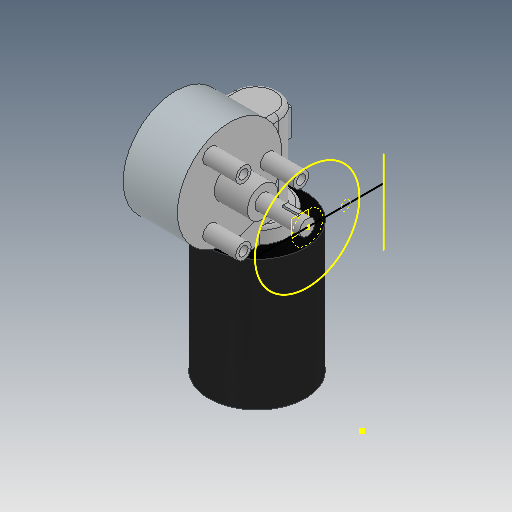
# Autodesk Inventor part: motor
Saved by Autodesk Inventor 2025.2 (Build 292293000, 293)
## iProperties
Created: 2024-10-20
Part Number: motor
Material: ABS Plastic
Document SubType Name: Modeling
Designer: email
Density: 1.06 g/cm^3
Appearance: Zinc
Author: email
Autodesk Inventor part; units mm, degrees
ref_plane "XZ Plane" through (0, 0, 0) normal (0, 1, 0) x (-1, 0, 0)
sketch "Sketch1" plane through (0, 0, 0) normal (0, 1, 0) x (-1, 0, 0)
  circle A0 centre (0, 0) radius 31.5
  circle A1 centre (0, 0) radius 20
  dimension "d0" = 63
  dimension "d29" = 40
  constraints: 2 centre point, 2 coincident
  measures "d0" diameter of A0
  measures "d29" diameter of A1
extrude "Extrusion1" add sketch "Sketch1" along normal blind 85 contours A0 | A1
sketch "Sketch2" plane through (0, 0, 0) normal (1, 0, 0) x (0, 1, 0)
  line L0 (0, -31.5) -> (85, -31.5) projected
  line L1 (0, -31.5) -> (0, 69.5)
  line L2 (0, 69.5) -> (166.6, 69.5)
  line L3 (166.6, 69.5) -> (166.6, 35.5)
  line L4 (166.6, 35.5) -> (132.6, 35.5)
  circle A0 centre (132.6, 35.5) radius 34
  circle A1 centre (132.6, 35.5) radius 25
  circle A2 centre (132.6, 10.5) radius 5
  circle A3 centre (132.6, 10.5) radius 3
  circle A4 centre (154.2506, 48) radius 5
  circle A5 centre (154.2506, 48) radius 3
  circle A6 centre (110.9494, 48) radius 5
  circle A7 centre (110.9494, 48) radius 3
  line L5 (85, -31.5) -> (85, 31.5) projected
  line L6 (85, 25.7084) -> (151.9419, 25.7084)
  line L7 (151.9419, 25.7084) -> (151.9419, -14.2916)
  line L8 (151.9419, -14.2916) -> (85, -14.2916)
  line L9 (85, -14.2916) -> (85, 25.7084)
  circle A8 centre (132.6, 35.5) radius 10
  circle A9 centre (132.6, 35.5) radius 5
  line L10 (85, 31.5) -> (85, 0)
  line L11 (85, 0) -> (100.814, 0)
  point P0 (0, 0)
  point P1 (151.9419, 7.5377)
  point P2 (134.9384, 1.5805)
  point P3 (130.2616, 1.5805)
  point P4 (100.0404, 25.7084)
  point P5 (92.907, 0)
  dimension "d8" = 50
  dimension "d3" = 101
  dimension "d4" = 166.6
  dimension "d5" = 34
  dimension "d6" = 34
  dimension "d7" = 68
  dimension "d9" = 10
  dimension "d10" = 6
  dimension "d13" = 360
  dimension "d21" = 20
  dimension "d22" = 10
  dimension "d26" = 40
  dimension "d49" = 69.5
  dimension "d50" = 35.5
  constraints: 20 end point, 9 centre point, 7 coincident, 3 horizontal, 3 point on line, 2 parallel, 2 perpendicular, 2 vertical, 1 midpoint, 1 vertical alignment, 15 other
  measures "d3" distance of L1.start L1.end
  measures "d4" distance of L1.end L2.end
  measures "d5" distance of L2.end L3.end
  measures "d6" distance of L3.end L4.end
  measures "d7" diameter of A0
  measures "d9" diameter of A2
  measures "d10" diameter of A3
  measures "d21" diameter of A8
  measures "d22" diameter of A9
  measures "d26" distance of L6.end L7.end
  measures "d49" distance between parallel lines of L2 L11
  measures "d50" distance from line of point (92.907, 0) L4
extrude "Extrusion2" add sketch "Sketch2" along normal mid plane 30 contours L5 L6 A0 L7 L8 | A0 L4 A1 A4 A6 L6 | A0 L7 A1 L4 | L6 A1 A2 L7 A0 | A1 L7 L6 A8 L4 | L4 A8 L6 A1 A6 A4 | L6 A8 L7 A1 A2 | A8 L6 | A4 A1 A5 | A1 A5 A4 | A6 A1 A7 | A1 A7 A6 | L6 A8 | A5 A1 | A1 A5 | A7 A1 | A1 A7 | A9
extrude "Extrusion3" add sketch "Sketch2" along normal blind 39.2 contours A8 L6 | A4 A1 A5 | A1 A5 A4 | A6 A1 A7 | A1 A7 A6 | A2 A1 A3 | A1 A3 A2 | L6 A8 | A5 A1 | A1 A5 | A7 A1 | A1 A7 | A3 A1 | A1 A3 | A9
extrude "Extrusion4" add sketch "Sketch2" along normal mid plane 35.35 contours A0 L4 A1 A4 A6 L6 | A0 L7 A1 L4 | L6 A1 A2 L7 A0 | A1 L7 L6 A8 L4 | L4 A8 L6 A1 A6 A4 | L6 A8 L7 A1 A2 | A8 L6 | A4 A1 A5 | A1 A5 A4 | A6 A1 A7 | A1 A7 A6 | A2 A1 A3 | A1 A3 A2 | L6 A8 | A5 A1 | A1 A5 | A7 A1 | A1 A7 | A3 A1 | A1 A3 | A9
extrude "Extrusion5" add sketch "Sketch2" along normal blind 68.2 contours A9
ref_plane "Work Plane1" through (-31.5, 0, 0) normal (1, 0, 0) x (0, 1, 0)
fillet "Fillet1" radius 15 2 edges at (15, 118.471, -14.2916) (-15, 118.471, -14.2916)
fillet "Fillet2" radius 3 3 edges at (15, 151.9419, 4.123) (-15, 151.9419, 4.123) (10.6066, 151.9419, -9.8982)
extrude "Extrusion6" add sketch "Sketch1" along normal blind 95 contours A1
fillet "Fillet3" radius 2 1 edges at (0, 95, -20)
ref_plane "Work Plane2" through (63.8, 132.6, 35.5) normal (1, 0, 0) x (0, 0, -1)
sketch "Sketch3" plane through (39.2, 154.2506, 48) normal (1, 0, 0) x (0, 0, -1)
  circle A0 centre (0, 0) radius 3
  circle A1 centre (37.5, -21.6506) radius 5 projected
  circle A2 centre (37.5, -21.6506) radius 3
  circle A3 centre (0, -43.3013) radius 5 projected
  circle A4 centre (0, -43.3013) radius 3
  point P0 (48, -154.2506)
  dimension "d33" = 6
  dimension "d34" = 6
  dimension "d35" = 6
  constraints: 3 centre point, 2 coincident
  measures "d33" diameter of A0
  measures "d34" diameter of A2
  measures "d35" diameter of A4
hole "Hole1" at (39.2, 154.2506, 48) at (39.2, 132.6, 10.5) at (39.2, 110.9494, 48) direction (-1, 0, 0) diameter 6 depth 10
sketch "Sketch4" plane through (63.8, 132.6, 35.5) normal (1, 0, 0) x (0, 0, -1)
  line L0 (-1.5, 3.8) -> (1.5, 3.8)
  line L1 (1.5, 3.8) -> (1.5, 6.2)
  line L2 (1.5, 6.2) -> (-1.5, 6.2)
  line L3 (-1.5, 6.2) -> (-1.5, 3.8)
  circle A0 centre (0, 0) radius 5 projected
  line L4 (-1.5, 3.8) -> (1.5, 6.2) construction
  line L5 (1.5, 3.8) -> (-1.5, 6.2) construction
  point P0 (35.5, -132.6)
  point P1 (0, 5)
  point P2 (-1.5, 4.7697)
  point P3 (1.5, 4.7697)
  dimension "d43" = 1.2
  dimension "d44" = 3
  constraints: 12 end point, 2 midpoint, 2 parallel, 1 horizontal, 1 perpendicular, 2 other
  measures "d43" distance from line of point (0, 5) L2
  measures "d44" distance of L1.end L2.end
extrude "Extrusion7" add sketch "Sketch4" against normal blind 9.9 contours L3 L2 L1 A0
ref_plane "Work Plane3" through (0, 0, -31.5) normal (0, 0, 1) x (1, 0, 0)
sketch "Sketch5" plane through (68.2, 132.6, 35.5) normal (1, 0, 0) x (0, 0, -1)
  circle A0 centre (0, 0) radius 10 construction
  circle A1 centre (25, 0) radius 3 construction
  line L0 (0, 0) -> (25, 0) construction
  line L1 (49.7916, -37.6) -> (49.7916, 16.3419) projected
  circle A2 centre (0, 0) radius 34 projected
  line L2 (49.7916, 0) -> (-34, 0)
  point P0 (35.5, -132.6)
  constraints: 4 end point, 1 horizontal, 1 horizontal alignment, 1 perpendicular, 1 point on line, 1 other
sketch "Sketch6" plane through (0, 0, 0) normal (1, 0, 0) x (0, 1, 0)
  line L0 (142.7057, -17.7741) -> (125.0557, -17.7741)
  line L1 (125.0557, -17.7741) -> (125.0557, -8.4301)
  line L2 (125.0557, -8.4301) -> (142.7057, -8.4301)
  line L3 (142.7057, -8.4301) -> (142.7057, -17.7741)
  circle A0 centre (132.6, 35.5) radius 34 projected
  point P0 (0, 0)
  point P1 (133.8807, 69.4759)
  point P2 (133.8807, -17.7741)
  dimension "d51" = 87.25
  dimension "d52" = 17.65
  constraints: 8 end point, 2 parallel, 1 horizontal, 1 midpoint, 1 perpendicular, 1 vertical alignment, 2 other
  measures "d51" distance from line of point (133.881, 69.476) L0
  measures "d52" distance between parallel lines of L1 L3
extrude "Extrusion8" add sketch "Sketch6" along normal mid plane 10 contours L0 L1 L2 L3
body "Solid1"
